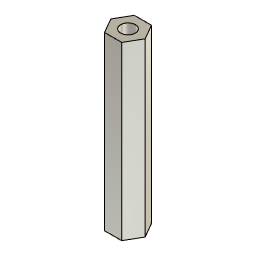
35mmスペーサー (Autodesk Fusion 360 design; units mm, degrees)
Autodesk Fusion 360 part; units mm, degrees
sketch "スケッチ1" plane through (0, 0, 0) normal (0, 0, 1) x (1, 0, 0)
  line L0 (3, 1.7321) -> (0, 3.4641)
  line L1 (0, 3.4641) -> (-3, 1.7321)
  line L2 (-3, 1.7321) -> (-3, -1.7321)
  line L3 (-3, -1.7321) -> (0, -3.4641)
  line L4 (0, -3.4641) -> (3, -1.7321)
  line L5 (3, -1.7321) -> (3, 1.7321)
  circle A0 centre (0, 0) radius 1.5
  constraint coincident A0.centre origin
extrude "押し出し1" add sketch "スケッチ1" along normal blind 35
sketch "スケッチ2" plane through (0, 0, 35) normal (0, 0, 1) x (-1, 0, 0)
  circle A0 centre (0, 0) radius 1.5
  line L0 (-3, 1.7321) -> (-3, -1.7321)
  line L1 (-3, -1.7321) -> (0, -3.4641)
  line L2 (0, -3.4641) -> (3, -1.7321)
  line L3 (3, -1.7321) -> (3, 1.7321)
  line L4 (3, 1.7321) -> (0, 3.4641)
  line L5 (0, 3.4641) -> (-3, 1.7321)
  line L6 (-3.5, 0) -> (-1.75, -3.0311)
  line L7 (-1.75, -3.0311) -> (1.75, -3.0311)
  line L8 (1.75, -3.0311) -> (3.5, 0)
  line L9 (3.5, 0) -> (1.75, 3.0311)
  line L10 (1.75, 3.0311) -> (-1.75, 3.0311)
  line L11 (-1.75, 3.0311) -> (-3.5, 0)
  constraint coincident A0.centre origin
extrude "押し出し2" add sketch "スケッチ2" along normal blind 4 contours L0 L1 L2 L3 L4 L5 L6 L7 L8 L9 L10 L11 | L0 L6 L11 | L5 L10 L11 | L1 L6 L7 | L4 L9 L10 | L2 L7 L8 | L3 L8 L9
extrude "押し出し3" cut 6 faces at (0, -3.1754, 35) (2.75, -1.5877, 35) (-2.75, -1.5877, 35) (-2.75, 1.5877, 35) (0, 3.1754, 35) (2.75, 1.5877, 35) along direction (0, 0, -1) blind 40
extrude "押し出し4" add 6 faces at (1.5833, 2.7424, 35) (3.1667, 0, 35) (-1.5833, 2.7424, 35) (1.5833, -2.7424, 35) (-1.5833, -2.7424, 35) (-3.1667, 0, 35) along direction (0, 0, -1) blind 35
extrude "押し出し5" cut 1 faces at (2.2005, 1.2273, 39) along direction (0, 0, -1) blind 4
